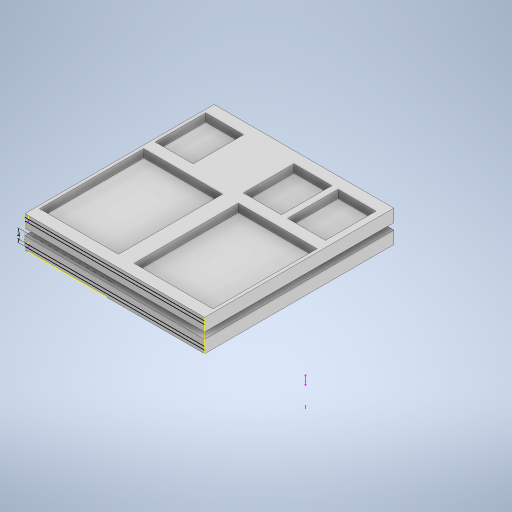
# Autodesk Inventor part: cotieni SD-micro SD versione2
Saved by Autodesk Inventor 2023 (Build 270158000, 158)
## iProperties
Created: 2023-07-25
Part Number: cotieni SD-micro SD versione2
Material: Generico
Document SubType Name: Modeling
Designer: Admin
Density: 1 g/cm^3
Appearance: Default
Author: Admin
Autodesk Inventor part; units mm, degrees
ref_plane "YZ Plane" through (0, 0, 0) normal (1, 0, 0) x (0, 1, 0)
ref_plane "XZ Plane" through (0, 0, 0) normal (0, 1, 0) x (-1, 0, 0)
ref_plane "XY Plane" through (0, 0, 0) normal (0, 0, 1) x (1, 0, 0)
sketch "Schizzo1" plane through (0, 0, 0) normal (0, 1, 0) x (-1, 0, 0)
  line L0 (28.5, 30) -> (-28.5, 30)
  line L1 (-28.5, 30) -> (-28.5, -30)
  line L2 (-28.5, -30) -> (28.5, -30)
  line L3 (28.5, -30) -> (28.5, 30)
  line L4 (0, 0) -> (0, -115.6454) construction
  line L5 (0, 0) -> (39.5796, 0) construction
  line L6 (27.5, 26.3333) -> (2.5, 26.3333)
  line L7 (2.5, 26.3333) -> (2.5, -6.6667)
  line L8 (2.5, -6.6667) -> (27.5, -6.6667)
  line L9 (27.5, -6.6667) -> (27.5, 26.3333)
  line L10 (28.5, 30) -> (28.5, 26.3333) construction
  line L11 (28.5, 26.3333) -> (27.5, 26.3333) construction
  line L12 (15.5, -10.3333) -> (15.5, -26.3333)
  line L13 (15.5, -26.3333) -> (27.5, -26.3333)
  line L14 (27.5, -26.3333) -> (27.5, -10.3333)
  line L15 (27.5, -10.3333) -> (15.5, -10.3333)
  line L16 (27.5, -6.6667) -> (27.5, -10.3333) construction
  line L17 (27.5, -10.3333) -> (28.5, -10.3333) construction
  line L18 (1.5, -10.3333) -> (1.5, -26.3333)
  line L19 (1.5, -26.3333) -> (13.5, -26.3333)
  line L20 (13.5, -10.3333) -> (1.5, -10.3333)
  line L21 (15.5, -10.3333) -> (13.5, -10.3333) construction
  line L22 (-2.5, -6.6667) -> (-27.5, -6.6667)
  line L23 (-27.5, -6.6667) -> (-27.5, 26.3333)
  line L24 (-27.5, 26.3333) -> (-2.5, 26.3333)
  line L25 (-2.5, 26.3333) -> (-2.5, -6.6667)
  line L26 (-14.5, -10.3333) -> (-14.5, -26.3333)
  line L27 (-14.5, -26.3333) -> (-26.5, -26.3333)
  line L28 (-26.5, -26.3333) -> (-26.5, -10.3333)
  line L29 (-26.5, -10.3333) -> (-14.5, -10.3333)
  line L30 (-0.5, -10.3333) -> (-0.5, -26.3333)
  line L31 (-12.5, -26.3333) -> (-12.5, -10.3333)
  line L32 (-12.5, -10.3333) -> (-0.5, -10.3333)
  line L33 (-0.5, -26.3333) -> (-12.5, -26.3333)
  line L34 (4.1, -0.1) -> (3.9, -0.1) construction
  line L35 (1.5, -10.3333) -> (-0.5, -10.3333) construction
  line L36 (-12.5, -10.3333) -> (-14.5, -10.3333) construction
  line L37 (2.5, 26.3333) -> (-2.5, 26.3333) construction
  line L38 (27.5, 30) -> (27.5, 0)
  line L39 (27.5, 0) -> (2.5, 0)
  line L40 (2.5, 0) -> (2.5, 30)
  line L41 (-27.5, 0) -> (-2.5, 0)
  line L42 (-2.5, 30) -> (-2.5, 0)
  line L43 (-2.5, 0) -> (-27.5, 0)
  line L44 (-27.5, 0) -> (-27.5, 30)
  line L45 (28, 30) -> (28, 26.3333) construction
  line L46 (27.5, -30) -> (27.5, -14)
  line L47 (27.5, -14) -> (15.5, -14)
  line L48 (15.5, -14) -> (15.5, -30)
  line L49 (27.5, -30) -> (27.5, -26.3333) construction
  line L50 (27.5, -26.3333) -> (28.5, -26.3333) construction
  line L51 (28, -26.3333) -> (28, -30) construction
  line L52 (15.5, -26.3333) -> (13.5, -26.3333) construction
  line L53 (-27.5, 26.3333) -> (-28.5, 26.3333) construction
  line L54 (13.5, -26.3333) -> (13.5, -10.3333)
  line L55 (1.5, -14) -> (1.5, -30)
  line L56 (13.5, -14) -> (1.5, -14)
  line L57 (13.5, -30) -> (13.5, -14)
  line L58 (-12.5, -14) -> (-12.5, -30)
  line L59 (-0.5, -14) -> (-12.5, -14)
  line L60 (-0.5, -30) -> (-0.5, -14)
  line L61 (-26.5, -14) -> (-26.5, -30)
  line L62 (-14.5, -14) -> (-26.5, -14)
  line L63 (-14.5, -30) -> (-14.5, -14)
  point P0 (0.4384, -30)
  point P1 (-4.1232, -30)
  dimension "d2" = 25
  dimension "d3" = 33
  dimension "d6" = 12
  dimension "d26" = 60
  dimension "d46" = 30
  dimension "d47" = 16
  dimension "d52" = 11.0796
  dimension "d61" = 57
  dimension "d62" = 2
  dimension "d63" = 16
  dimension "d66" = 14
  dimension "d71" = 5
  constraints: 130 end point, 22 perpendicular, 21 point on line, 16 parallel, 15 equal length, 7 horizontal, 4 collinear, 2 midpoint, 2 symmetric about line, 2 vertical, 23 other
  measures "d2" distance of L8.end L7.end
  measures "d3" distance of L7.end L6.end
  measures "d6" distance of L13.end L12.end
  measures "d26" distance of L2.end L0.start
  measures "d46" distance of L38.start L38.end
  measures "d47" distance of L46.start L46.end
  measures "d52" distance from line of L5.end L10
  measures "d61" distance of L1.end L2.end
  measures "d62" distance of L12.start L20.start
  measures "d63" distance of L19.end L54.end
  measures "d66" distance of L47.end L55.start
  measures "d71" distance of L6.end L25.start
extrude "Estrusione1" add sketch "Schizzo1" along normal mid plane 10 contours L3 L2 L46 L14 L15 L12 L48 L57 L54 L20 L18 L55 L60 L30 L32 L31 L58 L63 L26 L29 L28 L61 L1 L0 L44 L23 L22 L25 L42 L40 L7 L8 L9 L38 | L38 L6 L40 L0 | L2 L48 L13 L46 | L42 L24 L44 L0 | L2 L55 L19 L57 | L19 L18 L56 L54 | L2 L58 L33 L60 | L56 L18 L20 L54 | L61 L27 L63 L2
extrude "Estrusione2" add sketch "Schizzo1" along normal mid plane 5 contours L9 L39 L7 L6 | L9 L8 L7 L39 | L13 L12 L47 L14 | L25 L41 L23 L24 | L47 L12 L15 L14 | L25 L22 L23 L41 | L33 L31 L59 L30 | L28 L62 L26 L27 | L59 L31 L32 L30 | L28 L29 L26 L62
sketch "Schizzo3" plane through (-28.5, 5, 30) normal (0, 0, 1) x (1, 0, 0)
  line L0 (0, -10) -> (0, 0) construction
  line L1 (0, -5) -> (28.5, -5) construction
  line L2 (1, -10) -> (26, -10) projected
  line L3 (1, 0) -> (1, -2.5) projected
  line L4 (89, -2.5) -> (89, 0) projected
  line L5 (0, -5) -> (0, -9) construction
  line L6 (0, -5) -> (0, -8) construction
  line L7 (0, -8) -> (57, -8)
  line L8 (57, -10) -> (57, 0) projected
  line L9 (0, -9) -> (57, -9)
  line L10 (89, -9) -> (89, -8)
  line L11 (1, -9) -> (1, -8)
  line L12 (0, -2) -> (57, -2)
  line L13 (0, -1) -> (57, -1)
  line L14 (89, -1) -> (89, -2)
  line L15 (1, -1) -> (1, -2)
  point P0 (1, -7.5)
  dimension "d40" = 4
  dimension "d41" = 3
  constraints: 22 end point, 12 point on line, 8 symmetric about line, 2 perpendicular, 1 horizontal, 1 midpoint
  measures "d40" distance of L1.start L5.end
  measures "d41" distance of L1.start L6.end
extrude "Estrusione5" [suppressed]
sketch "Schizzo4" plane through (28.5, 5, -30) normal (0, 0, -1) x (-1, 0, 0)
  line L0 (89, -2) -> (89, -1) projected
  line L1 (89, -2) -> (89, -1)
  line L2 (89, -1) -> (1, -1) projected
  line L3 (89, -1) -> (1, -1)
  line L4 (1, -1) -> (1, -2) projected
  line L5 (1, -1) -> (1, -2)
  line L6 (1, -2) -> (89, -2) projected
  line L7 (1, -2) -> (89, -2)
  line L8 (89, -8) -> (1, -8) projected
  line L9 (1, -9) -> (89, -9) projected
  line L10 (89, -8) -> (89, -9)
  line L11 (89, -9) -> (1, -9)
  line L12 (1, -9) -> (1, -8)
  line L13 (1, -8) -> (89, -8)
  point P0 (28.5, -5)
  constraints: 16 end point, 4 perpendicular, 2 equal length, 2 vertical
extrude "Estrusione6" cut sketch "Schizzo4" against normal blind 2
extrude "Estrusione7" cut sketch "Schizzo1" along normal mid plane 2
extrude "Estrusione8" cut sketch "Schizzo1" along normal mid plane 1
